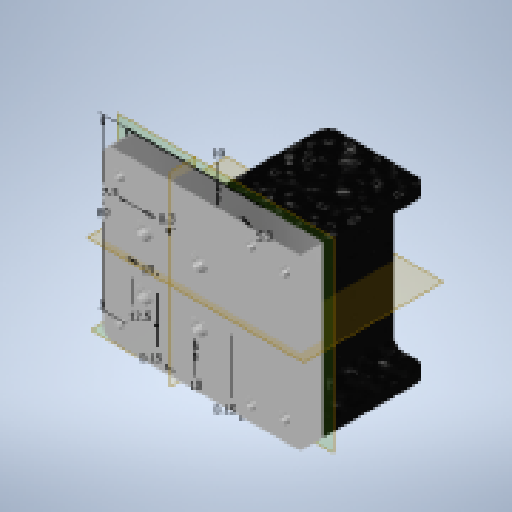
# Autodesk Inventor part: Soporte Actuador Lineal
Saved by Autodesk Inventor 2024 (Build 280153000, 153)
## iProperties
Created: 2023-12-10
Part Number: Soporte Actuador Lineal
Material: PET Plastic
Document SubType Name: Modeling
Designer: juanp
Density: 1.541 g/cm^3
Appearance: Black
Author: juanp
Autodesk Inventor part; units mm, degrees
ref_plane "YZ Plane" through (0, 0, 0) normal (1, 0, 0) x (0, 1, 0)
ref_plane "XZ Plane" through (0, 0, 0) normal (0, 1, 0) x (-1, 0, 0)
ref_plane "XY Plane" through (0, 0, 0) normal (0, 0, 1) x (1, 0, 0)
sketch "Sketch1" plane through (0, 0, 0) normal (0, 0, 1) x (1, 0, 0)
  line L0 (25, 39.4) -> (25, 0)
  line L1 (32, 0) -> (25, 0)
  line L2 (32, 0) -> (32, 39.4)
  line L3 (32, 39.4) -> (25, 39.4)
  circle A0 centre (29, 32.7) radius 2
  circle A1 centre (29, 6.7) radius 2
  line L4 (0, 0) -> (0, 39.4)
  line L5 (7, 0) -> (0, 0)
  line L6 (7, 0) -> (7, 39.4)
  line L7 (7, 39.4) -> (0, 39.4)
  circle A2 centre (3, 32.7) radius 2
  circle A3 centre (3, 6.7) radius 2
  line L8 (-1, 0) -> (-1, 39.4)
  line L9 (33, 39.4) -> (33, 0)
  line L10 (32.1572, 39.4) -> (32.1572, 50.4)
  line L11 (-0.2428, 50.4) -> (-0.2428, 39.4)
  line L12 (32.1572, 0) -> (32.1572, -11)
  line L13 (-0.2428, -11) -> (-0.2428, 0)
  line L14 (0, 39.4) -> (32, 39.4)
  line L15 (32, 39.4) -> (32, 0)
  line L16 (32, 0) -> (0, 0)
  line L17 (0, 0) -> (0, 39.4)
  line L18 (48, 59.7) -> (-16, 59.7)
  line L19 (-16, 59.7) -> (-16, -20.3)
  line L20 (-16, -20.3) -> (48, -20.3)
  line L21 (48, -20.3) -> (48, 59.7)
  line L22 (48, 59.7) -> (-16, -20.3) construction
  line L23 (-16, 59.7) -> (48, -20.3) construction
  line L24 (48, 49.7) -> (-16, 49.7) construction
  line L25 (48, -10.3) -> (-16, -10.3) construction
  line L26 (-8.5, -10.3) -> (40.5, -10.3) construction
  line L27 (40.5, -10.3) -> (40.5, 49.7) construction
  line L28 (40.5, 49.7) -> (-8.5, 49.7) construction
  line L29 (-8.5, 49.7) -> (-8.5, -10.3) construction
  line L30 (-8.5, -10.3) -> (40.5, 49.7) construction
  line L31 (40.5, -10.3) -> (-8.5, 49.7) construction
  circle A4 centre (40.5, 49.7) radius 2.65
  circle A5 centre (40.5, -10.3) radius 2.65
  circle A6 centre (-8.5, -10.3) radius 2.65
  circle A7 centre (-8.5, 49.7) radius 2.65
  circle A8 centre (3, 32.7) radius 2.3
  circle A9 centre (3, 6.7) radius 2.3
  circle A10 centre (29, 6.7) radius 2.3
  circle A11 centre (29, 32.7) radius 2.3
  line L32 (-13.65, 39.4) -> (-1.15, 39.4)
  line L33 (-1.15, 39.4) -> (-1.15, 0)
  line L34 (-1.15, 0) -> (-13.65, 0)
  line L35 (-13.65, 0) -> (-13.65, 39.4)
  line L36 (33.15, 39.4) -> (45.65, 39.4)
  line L37 (45.65, 39.4) -> (45.65, 0)
  line L38 (45.65, 0) -> (33.15, 0)
  line L39 (33.15, 0) -> (33.15, 39.4)
  point P0 (16, 19.7)
  dimension "d0" = 80
  dimension "d1" = 15
  dimension "d2" = 10
  dimension "d3" = 10
  dimension "d4" = 5.3
  dimension "d5" = 7.5
  dimension "d12" = 0.3
  dimension "d45" = 0.15
  dimension "d46" = 0.15
  dimension "d47" = 12.5
  constraints: 80 end point, 12 centre point, 10 parallel, 10 vertical, 9 horizontal, 8 coincident, 7 perpendicular, 6 equal radius, 5 collinear, 5 point on line, 4 midpoint, 30 other
  measures "d0" distance of L19.end L18.end
  measures "d1" distance between parallel lines of L8 L19
  measures "d2" distance between parallel lines of L18 L24
  measures "d3" distance between parallel lines of L20 L25
  measures "d4" diameter of A4
  measures "d5" distance between parallel lines of L29 L19
  measures "d12" radial gap between concentric circles of A2 A8
  measures "d45" distance between parallel lines of L9 L39
  measures "d46" distance between parallel lines of L33 L8
  measures "d47" distance between parallel lines of L35 L33
extrude "Extrusion1" add sketch "Sketch1" along normal blind 11 contours L3 L2 L1 L0 | L0 L16 L6 L14 | L6 L5 L4 L7 | L21 L20 L19 L18 | A4 | A5 | L32 L33 L34 L35 | L36 L37 L38 L39
sketch "Sketch2" plane through (0, 0, 11) normal (0, 0, 1) x (1, 0, 0)
  line L0 (48, 59.7) -> (-16, 59.7) projected
  line L1 (-16, 59.7) -> (-16, -20.3) projected
  line L2 (-16, -20.3) -> (48, -20.3) projected
  line L3 (48, -20.3) -> (48, 59.7) projected
  circle A0 centre (29, 32.7) radius 2.3 projected
  circle A1 centre (29, 6.7) radius 2.3 projected
  circle A2 centre (3, 6.7) radius 2.3 projected
  circle A3 centre (3, 32.7) radius 2.3 projected
  circle A4 centre (-8.5, 49.7) radius 2.65 projected
  circle A5 centre (-8.5, -10.3) radius 2.65 projected
  circle A6 centre (3, 32.7) radius 4
  circle A7 centre (3, 6.7) radius 4
  circle A8 centre (29, 6.7) radius 2.3 projected
  circle A9 centre (29, 6.7) radius 4
  circle A10 centre (29, 32.7) radius 4
  point P0 (-11, -20.3)
  dimension "d13" = 8
  constraints: 4 centre point, 4 coincident, 3 equal radius
  measures "d13" diameter of A6
extrude "Extrusion2" cut sketch "Sketch2" against normal blind 4 contours A0 | A1 | A2 | A3 | A6 | A7 | A9 | A10
ref_plane "Work Plane1" through (16, -15.3, 0) normal (1, 0, 0) x (0, 0, -1)
ref_plane "Work Plane2" through (-11, 19.7, 0) normal (0, 1, 0) x (1, 0, 0)
ref_plane "Work Plane3" through (-11, -20.3, 0) normal (0, -1, 0) x (1, 0, 0)
sketch "Sketch4" plane through (-16, -20.3, 0) normal (0, -1, 0) x (1, 0, 0)
  circle A0 centre (51, -43.975) radius 1.65 projected
  circle A1 centre (88, -19.325) radius 1.65 projected
  circle A2 centre (51, -19.325) radius 1.65 projected
  circle A3 centre (88, -43.975) radius 1.65 projected
  line L0 (51, -48.975) -> (88, -48.975) projected
  arc A4 (88, -48.975) -> (93, -43.975) centre (88, -43.975) ccw projected
  line L1 (93, -43.975) -> (93, -19.325) projected
  arc A5 (93, -19.325) -> (88, -14.325) centre (88, -19.325) ccw projected
  line L2 (88, -14.325) -> (51, -14.325) projected
  arc A6 (51, -14.325) -> (46, -19.325) centre (51, -19.325) ccw projected
  line L3 (46, -19.325) -> (46, -43.975) projected
  arc A7 (46, -43.975) -> (51, -48.975) centre (51, -43.975) ccw projected
  line L4 (64, 0) -> (64, 11) projected
  line L5 (64, 11) -> (93, 11)
  line L6 (93, 11) -> (93, -19.325)
  line L7 (46, -19.325) -> (46, 0)
  line L8 (42.7, 0) -> (47.3, 0) projected
  line L9 (0, 0) -> (64, 0) projected
  line L10 (64, 0) -> (64, 11) projected
  line L11 (0, 11) -> (64, 11) projected
  line L12 (0, 0) -> (0, 11) projected
  line L13 (47, -29.3406) -> (51, -27.0312) projected
  line L14 (51, -27.0312) -> (55, -29.3406) projected
  line L15 (55, -29.3406) -> (55, -33.9594) projected
  line L16 (55, -33.9594) -> (51, -36.2688) projected
  line L17 (51, -36.2688) -> (47, -33.9594) projected
  line L18 (47, -33.9594) -> (47, -29.3406) projected
  line L19 (84, -29.3406) -> (88, -27.0312) projected
  line L20 (88, -27.0312) -> (92, -29.3406) projected
  line L21 (92, -29.3406) -> (92, -33.9594) projected
  line L22 (92, -33.9594) -> (88, -36.2688) projected
  line L23 (88, -36.2688) -> (84, -33.9594) projected
  line L24 (84, -33.9594) -> (84, -29.3406) projected
  point P0 (16, 0)
  point P1 (57, 0)
  point P2 (57, 11)
  point P3 (46, 0)
  constraints: 6 end point, 1 horizontal, 1 perpendicular, 1 point on line, 1 vertical
extrude "Extrusion3" add sketch "Sketch4" against normal blind 5 contours A7 L3 A6 L2 A5 L1 A4 L0 | L7 L8 L9 L4 L5 L6 A5 L2 A6 | L13 L14 L15 L16 L17 L18 | L19 L20 L21 L22 L23 L24
sketch "Sketch9" plane through (-16, -15.3, 0) normal (0, 1, 0) x (1, 0, 0)
  line L0 (93, -11) -> (93, 43.975) projected
  arc A0 (93, 43.975) -> (88, 48.975) centre (88, 43.975) ccw projected
  line L1 (88, 48.975) -> (51, 48.975) projected
  arc A1 (51, 48.975) -> (46, 43.975) centre (51, 43.975) ccw projected
  line L2 (46, 43.975) -> (46, 0) projected
  line L3 (64, 0) -> (46, 0) projected
  circle A2 centre (51, 43.975) radius 1.65 projected
  circle A3 centre (88, 19.325) radius 1.65 projected
  circle A4 centre (51, 19.325) radius 1.65 projected
  circle A5 centre (88, 43.975) radius 1.65 projected
  circle A6 centre (51, 43.975) radius 1.65 projected
  line L4 (51, 40.7187) -> (48.18, 42.3469)
  line L5 (48.18, 42.3469) -> (48.18, 45.6031)
  line L6 (48.18, 45.6031) -> (51, 47.2313)
  line L7 (51, 47.2313) -> (53.82, 45.6031)
  line L8 (53.82, 45.6031) -> (53.82, 42.3469)
  line L9 (53.82, 42.3469) -> (51, 40.7187)
  line L10 (53.82, 17.6969) -> (51, 16.0687)
  line L11 (51, 16.0687) -> (48.18, 17.6969)
  line L12 (48.18, 17.6969) -> (48.18, 20.9531)
  line L13 (48.18, 20.9531) -> (51, 22.5813)
  line L14 (51, 22.5813) -> (53.82, 20.9531)
  line L15 (53.82, 20.9531) -> (53.82, 17.6969)
  line L16 (85.18, 20.9531) -> (88, 22.5813)
  line L17 (88, 22.5813) -> (90.82, 20.9531)
  line L18 (90.82, 20.9531) -> (90.82, 17.6969)
  line L19 (90.82, 17.6969) -> (88, 16.0687)
  line L20 (88, 16.0687) -> (85.18, 17.6969)
  line L21 (85.18, 17.6969) -> (85.18, 20.9531)
  line L22 (85.18, 45.6031) -> (88, 47.2313)
  line L23 (88, 47.2313) -> (90.82, 45.6031)
  line L24 (90.82, 45.6031) -> (90.82, 42.3469)
  line L25 (90.82, 42.3469) -> (88, 40.7187)
  line L26 (88, 40.7187) -> (85.18, 42.3469)
  line L27 (85.18, 42.3469) -> (85.18, 45.6031)
  line L28 (64, -11) -> (64, 0) projected
  line L29 (64, -11) -> (93, -11) projected
  point P0 (16, 0)
  dimension "d35" = 5.64
  constraints: 48 end point, 4 coincident, 4 vertical, 3 equal length, 52 other
  measures "d35" distance between parallel lines of L5 L8
extrude "Extrusion7" cut sketch "Sketch9" against normal blind 2.4 contours L4 L5 L6 L7 L8 L9 | L10 L11 L12 L13 L14 L15 | L16 L17 L18 L19 L20 L21 | L22 L23 L24 L25 L26 L27
mirror "Mirror1" about plane through (-11, 19.7, 0) normal (0, 1, 0) of "Extrusion3", "Extrusion7"
sketch "Sketch5" plane through (48, -15.3, 11) normal (1, 0, 0) x (0, 0, -1)
  line L0 (11, 0) -> (11, 70) projected
  line L1 (0, 0) -> (0, 70) projected
  line L2 (11, 0) -> (11, 70) projected
  line L3 (11, 70) -> (0, 70) projected
  line L4 (0, 0) -> (11, 0) projected
  point P0 (11, 15.3)
extrude "Extrusion4" add sketch "Sketch5" along normal up to surface (29 mm away)
sketch "Sketch7" plane through (0, 0, 0) normal (0, 0, -1) x (-1, 0, 0)
  circle A0 centre (8.5, -10.3) radius 2.65 projected
  circle A1 centre (8.5, 49.7) radius 2.65 projected
  circle A2 centre (-3, 32.7) radius 2.3 projected
  circle A3 centre (-3, 6.7) radius 2.3 projected
  circle A4 centre (-29, 6.7) radius 2.3 projected
  circle A5 centre (-29, 32.7) radius 2.3 projected
  line L0 (16, -20.3) -> (-30, -20.3) projected
  line L1 (16, 59.7) -> (16, -20.3) projected
  line L2 (-30, 59.7) -> (16, 59.7) projected
  circle A6 centre (-69.5, -10.3) radius 2.65
  circle A7 centre (-69.5, 49.7) radius 2.65
  circle A8 centre (8.5, -10.3) radius 2.65 projected
  line L3 (-30, 59.7) -> (-30, 54.7) projected
  line L4 (-77, 54.7) -> (-30, 54.7) projected
  line L5 (-77, 54.7) -> (-77, -15.3) projected
  line L6 (-77, -15.3) -> (-30, -15.3) projected
  line L7 (-30, -15.3) -> (-30, -20.3) projected
  point P0 (0, 0)
  constraints: 2 centre point, 2 equal radius
extrude "Extrusion5" cut sketch "Sketch7" against normal through all contours A6 | A7
sketch "Sketch8" plane through (0, 0, 0) normal (0, 0, -1) x (-1, 0, 0)
  line L0 (-77, -15.3) -> (-30, -15.3) projected
  line L1 (-46, -15.3) -> (-61, -15.3)
  line L2 (-61, -15.3) -> (-61, 54.7)
  line L3 (-61, 54.7) -> (-46, 54.7)
  line L4 (-46, 54.7) -> (-46, -15.3)
  line L5 (-72, 54.7) -> (-35, 54.7) projected
  point P0 (0, 0)
  point P1 (-53.5, 54.7)
  dimension "d23" = 15
  constraints: 8 end point, 2 midpoint, 2 parallel, 1 horizontal, 1 perpendicular, 1 point on line
  measures "d23" distance between parallel lines of L2 L4
extrude "Extrusion6" add sketch "Sketch8" along normal up to surface (48.975 mm away)
chamfer "Chamfer1" distance 3 angle 45 4 edges at (46, -15.3, -24.4875) (61, -15.3, -24.4875) (61, 54.7, -24.4875) (46, 54.7, -24.4875)
fillet "Fillet2" radius 5 2 edges at (-16, 59.7, 5.5) (-16, -20.3, 5.5)
ref_plane "Work Plane4" through (0, 0, 0) normal (0, 0, -1) x (-1, 0, 0)
extrude "Extrusion9" add sketch "Sketch1" against normal blind 12.5 contours L32 L33 L34 L35 | L36 L37 L38 L39
chamfer "Chamfer2" distance 6.25 angle 45 2 edges at (-13.65, 19.7, -12.5) (45.65, 19.7, -12.5)
body "Solid1"
body "Solid3"
